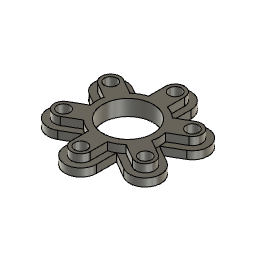
Model 22 (Autodesk Fusion 360 design; units mm, degrees)
Autodesk Fusion 360 part; units mm, degrees
sketch "Sketch1" plane through (0, 0, 0) normal (0, 0, 1) x (1, 0, 0)
  circle A0 centre (0, 0) radius 16
  circle A1 centre (0, 0) radius 30 construction
  line L0 (0, 0) -> (0, 30) construction
  line L1 (0, 0) -> (30, 0) construction
  line L2 (0, 0) -> (-30, 0) construction
  line L3 (0, 0) -> (0, -30) construction
  circle A2 centre (0, 30) radius 4
  line L4 (0, 30) -> (10, 30) construction
  line L5 (10, 30) -> (10, 17.3205)
  line L6 (0, 30) -> (-10, 30) construction
  line L7 (-10, 30) -> (-10, 17.3205)
  line L8 (-6, 30) -> (-6, 19.0788)
  line L9 (6, 30) -> (6, 19.0788)
  arc A3 (5.9699, 29.4) -> (-5.9699, 29.4) centre (0, 30) ccw
  arc A4 (9.8601, 28.3333) -> (-9.8601, 28.3333) centre (0, 30) ccw
  line L10 (-30.9808, 6.3397) -> (-20, 0)
  arc A5 (-19.6073, 22.7058) -> (-29.4675, 5.6275) centre (-25.9808, 15) ccw
  line L11 (-20.9808, 23.6603) -> (-10, 17.3205)
  line L12 (-22.9808, 20.1962) -> (-13.5227, 14.7355)
  line L13 (-28.9808, 9.8038) -> (-19.5227, 4.3432)
  arc A6 (-22.4762, 19.8701) -> (-28.4461, 9.5299) centre (-25.9808, 15) ccw
  circle A7 centre (-25.9808, 15) radius 4
  line L14 (-20.9808, -23.6603) -> (-10, -17.3205)
  arc A8 (-29.4675, -5.6275) -> (-19.6073, -22.7058) centre (-25.9808, -15) ccw
  line L15 (-30.9808, -6.3397) -> (-20, 0)
  line L16 (-28.9808, -9.8038) -> (-19.5227, -4.3432)
  line L17 (-22.9808, -20.1962) -> (-13.5227, -14.7355)
  arc A9 (-28.4461, -9.5299) -> (-22.4762, -19.8701) centre (-25.9808, -15) ccw
  circle A10 centre (-25.9808, -15) radius 4
  line L18 (10, -30) -> (10, -17.3205)
  arc A11 (-9.8601, -28.3333) -> (9.8601, -28.3333) centre (0, -30) ccw
  line L19 (-10, -30) -> (-10, -17.3205)
  line L20 (-6, -30) -> (-6, -19.0788)
  line L21 (6, -30) -> (6, -19.0788)
  arc A12 (-5.9699, -29.4) -> (5.9699, -29.4) centre (0, -30) ccw
  circle A13 centre (0, -30) radius 4
  line L22 (30.9808, -6.3397) -> (20, 0)
  arc A14 (19.6073, -22.7058) -> (29.4675, -5.6275) centre (25.9808, -15) ccw
  line L23 (20.9808, -23.6603) -> (10, -17.3205)
  line L24 (22.9808, -20.1962) -> (13.5227, -14.7355)
  line L25 (28.9808, -9.8038) -> (19.5227, -4.3432)
  arc A15 (22.4762, -19.8701) -> (28.4461, -9.5299) centre (25.9808, -15) ccw
  circle A16 centre (25.9808, -15) radius 4
  line L26 (20.9808, 23.6603) -> (10, 17.3205)
  arc A17 (29.4675, 5.6275) -> (19.6073, 22.7058) centre (25.9808, 15) ccw
  line L27 (30.9808, 6.3397) -> (20, 0)
  line L28 (28.9808, 9.8038) -> (19.5227, 4.3432)
  line L29 (22.9808, 20.1962) -> (13.5227, 14.7355)
  arc A18 (28.4461, 9.5299) -> (22.4762, 19.8701) centre (25.9808, 15) ccw
  circle A19 centre (25.9808, 15) radius 4
  arc A20 (-6, 19.0788) -> (-13.5227, 14.7355) centre (0, 0) ccw
  arc A21 (13.5227, 14.7355) -> (6, 19.0788) centre (0, 0) ccw
  arc A22 (19.5227, -4.3432) -> (19.5227, 4.3432) centre (0, 0) ccw
  arc A23 (6, -19.0788) -> (13.5227, -14.7355) centre (0, 0) ccw
  arc A24 (-19.5227, 4.3432) -> (-19.5227, -4.3432) centre (0, 0) ccw
  arc A25 (-13.5227, -14.7355) -> (-6, -19.0788) centre (0, 0) ccw
  dimension "d1" = 32
  dimension "d2" = 40
  dimension "d3" = 60
  dimension "d4" = 8
  dimension "d5" = 12
  dimension "d6" = 20
  dimension "d8" = 360
  constraint coincident A0.centre A1.centre
  constraint concentric A0 A24
  constraint concentric A1 A24
  constraint coincident A1 L0.end
  constraint vertical L0
  constraint coincident A1 L1.end
  constraint perpendicular L0 L1
  constraint coincident A1 L2.end
  constraint parallel L1 L2
  constraint coincident A1 L3.end
  constraint perpendicular L2 L3
  constraint coincident L0.end A2.centre
  constraint concentric A2 A3
  constraint concentric A3 A4
  constraint coincident L4.end A4
  constraint horizontal L4
  constraint coincident L5.end A24
  constraint tangent L5 A4
  constraint coincident L6.end A4
  constraint tangent A1 L6
  constraint horizontal L6
  constraint coincident L7.end A24
  constraint perpendicular L6 L7
  constraint coincident L8.start A3
  constraint coincident L6 L8.start
  constraint coincident L8.end A24
  constraint tangent L8 A3
  constraint coincident L9.start A3
  constraint coincident L4 L9.start
  constraint tangent L9 A3
  constraint coincident A1 A3.start
  constraint coincident A1 A3.end
  constraint coincident A1 A4.start
  constraint coincident A1 A4.end
  constraint concentric A20 A24
  constraint concentric A21 A24
  constraint concentric A22 A24
  constraint concentric A23 A24
  constraint concentric A24 A25
  measures "d1" diameter of A0
  measures "d2" diameter of A24
  measures "d3" diameter of A1
  measures "d4" diameter of A2
  measures "d5" diameter of A3
  measures "d6" diameter of A4
extrude "Extrude1" add sketch "Sketch1" along normal blind 10 contours L8 L9 A3 L12 L13 A6 L16 L17 A9 L20 L21 A12 L24 L25 A15 L28 L29 A18 A20 A21 A22 A23 A24 A25 makes body 1
extrude "Extrude2" add sketch "Sketch1" along normal blind 5 separate body contours L5 L7 L8 L9 A3 A4 A20 A21 | L26 A17 L27 L28 L29 A18 A21 A22 | L10 A5 L11 L12 L13 A6 A20 A24 | L22 A14 L23 L24 L25 A15 A22 A23 | L14 A8 L15 L16 L17 A9 A24 A25 | L18 A11 L19 L20 L21 A12 A23 A25 makes body 2 at (-26.4947, 6.8289, 0)
